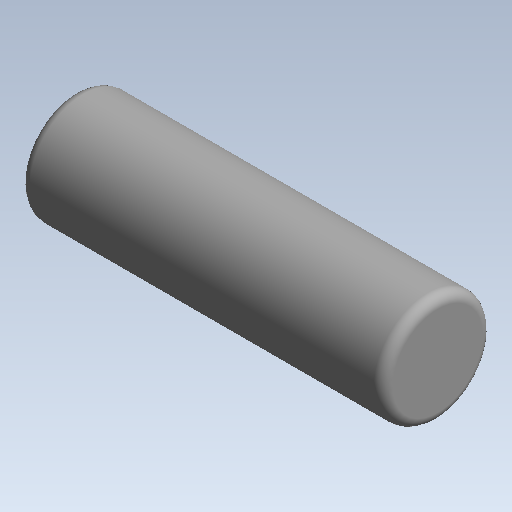
# Autodesk Inventor part: HK0609FMRO
Saved by Autodesk Inventor 2021.3 (Build 253353010, 353A)
## iProperties
Part Number: HK0609FMRO
Material: 一般
Catalog Web Link: www.cadenas.de
Description: Needle Roller Shell Bearings open-ended RO-
Vendor: NTN
Document SubType Name: Modeling
Designer: partserver
Manufacturer: NTN
Mass: 0.0088012 g
Surface Area: 0.265411 cm^2
Volume: 0.0088012 cm^3
Density: 1 g/cm^3
Appearance: PSOLRGB-192-192-192
Category: PARTsolutions
Company: NTN
PSOL_IDENT_0: {$CADENAS_DATA\23d-libs\ntn\needle_roler_bearings\needle_roller_shell_bearings_open_ended_ro.prj},19
PSOL_IDENT_1: 6 {VTYP=3D},{NB=HK0609FMRO},{LINA=HK0609FMRO},{NN=Needle Roller Shell Bearings open-ended RO},{DATE=
PSOL_IDENT_2: 23.10.2020 01:12:34},{GEOMDATE=20.04.2020 08:34:27},{VERSION=},{LINEID=40},{WBVAR=},{WBNUMERIC=}  {N
PSOL_IDENT_3: B=HK0609FMRO},{LINA=HK0609FMRO},{KT=DUMMY},{FW=6},{D=10.0},{C=9},{ORDER=HK0609FM},{CR=2920},{COR=259
PSOL_IDENT_4: 0},{CRF=298},{CORF=264},{LSG=25000},{LSO=37000},{MASS=0.0022},{IT=-},{RT=1.6},{VER=1},{T=0.500},{DW=
PSOL_IDENT_5: 1.500},{LW=5.000},{NR=9.000},{CID=6.750},{CD=8.250},{CW=7.600},{SD=6.300}
NB: HK0609FMRO
NN: Needle Roller Shell Bearings open-ended RO
NBSYN: $ORDER.RO
LINA: HK0609FMRO
CATALOG: NTN Corporation
FW: 6
D: 10
C: 9
ORDER: HK0609FM
CR: 2920
COR: 2590
CRF: 298
CORF: 264
LSG: 25000
LSO: 37000
MASS: 0.0022
IT: -
RT: 1.6
VER: 1
SUPPLIER: NTN
ARTICLENO: HK0609FMRO
BOMINFO: HK0609FMRO
CREATOR: CADENAS GmbH
Title: HK0609FMRO
Author: Cadenas PARTsolutions
Autodesk Inventor part; units mm, degrees
sketch "Sketch_1" plane through (0, 0, 0) normal (0, 0, 1) x (1, 0, 0)
  line L0 (2.5, 0) -> (-2.5, 0)
  line L1 (-2.5, 0) -> (-2.5, 0.6167)
  arc A0 (-2.3667, 0.75) -> (-2.5, 0.6167) centre (-2.3667, 0.6167) ccw
  line L2 (-2.3667, 0.75) -> (2.3667, 0.75)
  arc A1 (2.5, 0.6167) -> (2.3667, 0.75) centre (2.3667, 0.6167) ccw
  line L3 (2.5, 0.6167) -> (2.5, 0)
  line L4 (2.5, 0) -> (-2.5, 0)
  constraints: 10 end point, 4 point on circle, 2 centre point
revolve "Revolution1" add sketch "Sketch_1" angle 360 about axis through (2.5, 0, 0) along (1, 0, 0)
ref_plane "IP_1_XY" through (0, 0, 0) normal (1, 0, 0) x (0, 0, -1)
ref_plane "IP_1_YZ" through (0, 0, 0) normal (0, 0, -1) x (0, 1, 0)
ref_plane "IP_1_ZX" through (0, 0, 0) normal (0, 1, 0) x (1, 0, 0)
body "Solid1"
